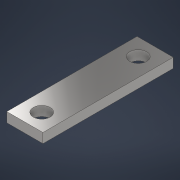
# Autodesk Inventor part: Планка
Saved by Autodesk Inventor 2021 (Build 250183000, 183)
## iProperties
Created: 2022-05-01
Part Number: Планка
Material: Stainless Steel
Document SubType Name: Modeling
Designer: DuctopwH
Density: 8 g/cm^3
Appearance: Semi-Polished
Author: DuctopwH
Autodesk Inventor part; units mm, degrees
ref_plane "YZ Plane" through (0, 0, 0) normal (1, 0, 0) x (0, 1, 0)
ref_plane "XZ Plane" through (0, 0, 0) normal (0, 1, 0) x (-1, 0, 0)
ref_plane "XY Plane" through (0, 0, 0) normal (0, 0, 1) x (1, 0, 0)
sketch "Sketch1" plane through (0, 0, 0) normal (0, 1, 0) x (-1, 0, 0)
  line L0 (-7.5, 27) -> (7.5, 27)
  line L1 (7.5, 27) -> (7.5, -27)
  line L2 (7.5, -27) -> (-7.5, -27)
  line L3 (-7.5, -27) -> (-7.5, 27)
  line L4 (-7.5, 27) -> (7.5, -27) construction
  line L5 (7.5, 27) -> (-7.5, -27) construction
  circle A0 centre (0, -20) radius 3.5
  circle A1 centre (0, 20) radius 3.5
  line L6 (7.5, 0) -> (0, 0)
  point P0 (0, 0)
  dimension "d0" = 7
  dimension "d1" = 15
  dimension "d2" = 54
  dimension "d3" = 40
  constraints: 14 end point, 4 midpoint, 2 centre point, 2 horizontal, 2 parallel, 1 perpendicular, 1 vertical alignment, 1 other
  measures "d0" diameter of A0
  measures "d1" distance between parallel lines of L3 L1
  measures "d2" distance between parallel lines of L0 L2
  measures "d3" distance of A1.centre A0.centre
extrude "Extrusion1" add sketch "Sketch1" along normal mid plane 4
body "Solid1"
